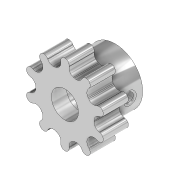
# Autodesk Inventor part: 4th Axis Main Drive Gear
Saved by Autodesk Inventor 2020 (Build 240168000, 168)
## iProperties
Created: 2021-06-28
Part Number: 4th Axis Main Drive Gear
Material: Generic
Document SubType Name: Modeling
Designer: Coy
Density: 1 g/cm^3
Appearance: Chrome - Polished
Author: Coy
Autodesk Inventor part; units mm, degrees
ref_plane "YZ Plane" through (0, 0, 0) normal (1, 0, 0) x (0, 1, 0)
ref_plane "XZ Plane" through (0, 0, 0) normal (0, 1, 0) x (-1, 0, 0)
ref_plane "XY Plane" through (0, 0, 0) normal (0, 0, 1) x (1, 0, 0)
sketch "Sketch4" plane through (0, 0, 0) normal (0, 0, 1) x (1, 0, 0)
  circle A0 centre (0, 0) radius 2.5
  circle A1 centre (0, 0) radius 8.2 construction
  arc A2 (1.0386, 6.9958) -> (-1.0386, 6.9958) centre (0, 7.15) ccw
  arc A3 (-1.7552, 5.7375) -> (-1.0238, 6.8958) centre (-2.0624, 6.7416) ccw
  arc A4 (1.0238, 6.8958) -> (1.7552, 5.7375) centre (2.0624, 6.7416) ccw
  line L0 (1.0238, 6.8958) -> (1.0386, 6.9958)
  line L1 (-1.0238, 6.8958) -> (-1.0386, 6.9958)
  line L2 (0, 0) -> (0, 6.1) construction
  line L3 (0, 8.2) -> (0, 9.5985) construction
  arc A5 (-3.2718, 6.2702) -> (-4.9523, 5.0492) centre (-4.2027, 5.7845) ccw
  line L4 (-4.8815, 4.9771) -> (-4.9523, 5.0492)
  arc A6 (-4.7924, 3.6101) -> (-4.8815, 4.9771) centre (-5.6311, 4.2418) ccw
  line L5 (-3.225, 6.1806) -> (-3.2718, 6.2702)
  arc A7 (-3.225, 6.1806) -> (-1.9524, 5.6734) centre (-2.2941, 6.6663) ccw
  arc A8 (-6.3325, 3.1496) -> (-6.9744, 1.174) centre (-6.8001, 2.2095) ccw
  line L6 (-6.8746, 1.1573) -> (-6.9744, 1.174)
  arc A9 (-5.9991, 0.1037) -> (-6.8746, 1.1573) centre (-7.0489, 0.1218) ccw
  line L7 (-6.2419, 3.1046) -> (-6.3325, 3.1496)
  arc A10 (-6.2419, 3.1046) -> (-4.9143, 3.4423) centre (-5.7743, 4.0447) ccw
  arc A11 (-6.9744, -1.174) -> (-6.3325, -3.1496) centre (-6.8001, -2.2095) ccw
  line L8 (-6.2419, -3.1046) -> (-6.3325, -3.1496)
  arc A12 (-4.9143, -3.4423) -> (-6.2419, -3.1046) centre (-5.7743, -4.0447) ccw
  line L9 (-6.8746, -1.1573) -> (-6.9744, -1.174)
  arc A13 (-6.8746, -1.1573) -> (-5.9991, -0.1037) centre (-7.0489, -0.1218) ccw
  arc A14 (-4.9523, -5.0492) -> (-3.2718, -6.2702) centre (-4.2027, -5.7845) ccw
  line L10 (-3.225, -6.1806) -> (-3.2718, -6.2702)
  arc A15 (-1.9524, -5.6734) -> (-3.225, -6.1806) centre (-2.2941, -6.6663) ccw
  line L11 (-4.8815, -4.9771) -> (-4.9523, -5.0492)
  arc A16 (-4.8815, -4.9771) -> (-4.7924, -3.6101) centre (-5.6311, -4.2418) ccw
  arc A17 (-1.0386, -6.9958) -> (1.0386, -6.9958) centre (0, -7.15) ccw
  line L12 (1.0238, -6.8958) -> (1.0386, -6.9958)
  arc A18 (1.7552, -5.7375) -> (1.0238, -6.8958) centre (2.0624, -6.7416) ccw
  line L13 (-1.0238, -6.8958) -> (-1.0386, -6.9958)
  arc A19 (-1.0238, -6.8958) -> (-1.7552, -5.7375) centre (-2.0624, -6.7416) ccw
  arc A20 (3.2718, -6.2702) -> (4.9523, -5.0492) centre (4.2027, -5.7845) ccw
  line L14 (4.8815, -4.9771) -> (4.9523, -5.0492)
  arc A21 (4.7924, -3.6101) -> (4.8815, -4.9771) centre (5.6311, -4.2418) ccw
  line L15 (3.225, -6.1806) -> (3.2718, -6.2702)
  arc A22 (3.225, -6.1806) -> (1.9524, -5.6734) centre (2.2941, -6.6663) ccw
  arc A23 (6.3325, -3.1496) -> (6.9744, -1.174) centre (6.8001, -2.2095) ccw
  line L16 (6.8746, -1.1573) -> (6.9744, -1.174)
  arc A24 (5.9991, -0.1037) -> (6.8746, -1.1573) centre (7.0489, -0.1218) ccw
  line L17 (6.2419, -3.1046) -> (6.3325, -3.1496)
  arc A25 (6.2419, -3.1046) -> (4.9143, -3.4423) centre (5.7743, -4.0447) ccw
  arc A26 (6.9744, 1.174) -> (6.3325, 3.1496) centre (6.8001, 2.2095) ccw
  line L18 (6.2419, 3.1046) -> (6.3325, 3.1496)
  arc A27 (4.9143, 3.4423) -> (6.2419, 3.1046) centre (5.7743, 4.0447) ccw
  line L19 (6.8746, 1.1573) -> (6.9744, 1.174)
  arc A28 (6.8746, 1.1573) -> (5.9991, 0.1037) centre (7.0489, 0.1218) ccw
  arc A29 (4.9523, 5.0492) -> (3.2718, 6.2702) centre (4.2027, 5.7845) ccw
  line L20 (3.225, 6.1806) -> (3.2718, 6.2702)
  arc A30 (1.9524, 5.6734) -> (3.225, 6.1806) centre (2.2941, 6.6663) ccw
  line L21 (4.8815, 4.9771) -> (4.9523, 5.0492)
  arc A31 (4.8815, 4.9771) -> (4.7924, 3.6101) centre (5.6311, 4.2418) ccw
  arc A32 (-1.7552, 5.7375) -> (-1.9524, 5.6734) centre (0, 0) ccw
  arc A33 (1.9524, 5.6734) -> (1.7552, 5.7375) centre (0, 0) ccw
  arc A34 (4.9143, 3.4423) -> (4.7924, 3.6101) centre (0, 0) ccw
  arc A35 (5.9991, -0.1037) -> (5.9991, 0.1037) centre (0, 0) ccw
  arc A36 (4.7924, -3.6101) -> (4.9143, -3.4423) centre (0, 0) ccw
  arc A37 (1.7552, -5.7375) -> (1.9524, -5.6734) centre (0, 0) ccw
  arc A38 (-1.9524, -5.6734) -> (-1.7552, -5.7375) centre (0, 0) ccw
  arc A39 (-4.9143, -3.4423) -> (-4.7924, -3.6101) centre (0, 0) ccw
  arc A40 (-4.7924, 3.6101) -> (-4.9143, 3.4423) centre (0, 0) ccw
  arc A41 (-5.9991, 0.1037) -> (-5.9991, -0.1037) centre (0, 0) ccw
  point P0 (-4.8198, 6.6339)
  point P1 (-7.7987, 2.5339)
  point P2 (-7.7987, -2.5339)
  point P3 (-4.8198, -6.6339)
  point P4 (0, -8.2)
  point P5 (4.8198, -6.6339)
  point P6 (7.7987, -2.5339)
  point P7 (7.7987, 2.5339)
  point P8 (4.8198, 6.6339)
  dimension "d19" = 5
  dimension "d20" = 16.4
  dimension "d22" = 2.1
  dimension "d23" = 2.1
  dimension "d24" = 2.1
  dimension "d27" = 360
  constraints: 90 point on circle, 44 end point, 42 centre point, 20 line through centre, 5 tangent, 2 coincident, 2 vertical, 151 other
  measures "d19" diameter of A0
  measures "d20" diameter of A1
  measures "d22" diameter of A2
  measures "d23" diameter of A4
  measures "d24" diameter of A3
extrude "Extrusion4" add sketch "Sketch4" along normal blind 5
sketch "Sketch5" plane through (0, 0, 0) normal (0, 0, -1) x (-1, 0, 0)
  circle A0 centre (0, 0) radius 2.5
  circle A1 centre (0, 0) radius 5.5
  dimension "d31" = 3
  constraints: 2 centre point, 1 coincident, 1 other
  measures "d31" radial gap between concentric circles of A0 A1
extrude "Extrusion5" add sketch "Sketch5" along normal blind 5
sketch "Sketch6" plane through (0, 0, 0) normal (1, 0, 0) x (0, 1, 0)
  line L0 (5.5, 0) -> (5.5, -5) projected
  line L1 (5.5, -2.5) -> (-5.5, -2.5) construction
  line L2 (-5.5, 0) -> (-5.5, -5) construction
  circle A0 centre (0, -2.5) radius 0.95
  point P0 (0, 0)
  dimension "d34" = 1.9
  constraints: 3 midpoint, 2 end point, 1 centre point
  measures "d34" diameter of A0
extrude "Extrusion6" cut sketch "Sketch6" against normal through all both and the other way through all
sketch "Sketch7" plane through (0, 0, 5) normal (0, 0, 1) x (1, 0, 0)
  arc A0 (-6.3325, 3.1496) -> (-6.9744, 1.174) centre (-6.8001, 2.2095) ccw projected
  line L0 (-6.9744, 1.174) -> (-6.8746, 1.1573) projected
  arc A1 (-5.9991, 0.1037) -> (-6.8746, 1.1573) centre (-7.0489, 0.1218) ccw projected
  arc A2 (-5.9991, 0.1037) -> (-5.9991, -0.1037) centre (0, 0) ccw projected
  arc A3 (-6.8746, -1.1573) -> (-5.9991, -0.1037) centre (-7.0489, -0.1218) ccw projected
  line L1 (-6.8746, -1.1573) -> (-6.9744, -1.174) projected
  arc A4 (-6.9744, -1.174) -> (-6.3325, -3.1496) centre (-6.8001, -2.2095) ccw projected
  line L2 (-6.3325, -3.1496) -> (-6.2419, -3.1046) projected
  arc A5 (-4.9143, -3.4423) -> (-6.2419, -3.1046) centre (-5.7743, -4.0447) ccw projected
  arc A6 (-4.9143, -3.4423) -> (-4.7924, -3.6101) centre (0, 0) ccw projected
  arc A7 (-4.8815, -4.9771) -> (-4.7924, -3.6101) centre (-5.6311, -4.2418) ccw projected
  line L3 (-4.8815, -4.9771) -> (-4.9523, -5.0492) projected
  arc A8 (-4.9523, -5.0492) -> (-3.2718, -6.2702) centre (-4.2027, -5.7845) ccw projected
  line L4 (-3.2718, -6.2702) -> (-3.225, -6.1806) projected
  arc A9 (-1.9524, -5.6734) -> (-3.225, -6.1806) centre (-2.2941, -6.6663) ccw projected
  arc A10 (-1.9524, -5.6734) -> (-1.7552, -5.7375) centre (0, 0) ccw projected
  arc A11 (-1.0238, -6.8958) -> (-1.7552, -5.7375) centre (-2.0624, -6.7416) ccw projected
  line L5 (-1.0238, -6.8958) -> (-1.0386, -6.9958) projected
  arc A12 (-1.0386, -6.9958) -> (1.0386, -6.9958) centre (0, -7.15) ccw projected
  line L6 (1.0386, -6.9958) -> (1.0238, -6.8958) projected
  arc A13 (1.7552, -5.7375) -> (1.0238, -6.8958) centre (2.0624, -6.7416) ccw projected
  arc A14 (1.7552, -5.7375) -> (1.9524, -5.6734) centre (0, 0) ccw projected
  arc A15 (3.225, -6.1806) -> (1.9524, -5.6734) centre (2.2941, -6.6663) ccw projected
  line L7 (3.225, -6.1806) -> (3.2718, -6.2702) projected
  arc A16 (3.2718, -6.2702) -> (4.9523, -5.0492) centre (4.2027, -5.7845) ccw projected
  line L8 (4.9523, -5.0492) -> (4.8815, -4.9771) projected
  arc A17 (4.7924, -3.6101) -> (4.8815, -4.9771) centre (5.6311, -4.2418) ccw projected
  arc A18 (4.7924, -3.6101) -> (4.9143, -3.4423) centre (0, 0) ccw projected
  arc A19 (6.2419, -3.1046) -> (4.9143, -3.4423) centre (5.7743, -4.0447) ccw projected
  line L9 (6.2419, -3.1046) -> (6.3325, -3.1496) projected
  arc A20 (6.3325, -3.1496) -> (6.9744, -1.174) centre (6.8001, -2.2095) ccw projected
  line L10 (6.9744, -1.174) -> (6.8746, -1.1573) projected
  arc A21 (5.9991, -0.1037) -> (6.8746, -1.1573) centre (7.0489, -0.1218) ccw projected
  arc A22 (5.9991, -0.1037) -> (5.9991, 0.1037) centre (0, 0) ccw projected
  arc A23 (6.8746, 1.1573) -> (5.9991, 0.1037) centre (7.0489, 0.1218) ccw projected
  line L11 (6.8746, 1.1573) -> (6.9744, 1.174) projected
  arc A24 (6.9744, 1.174) -> (6.3325, 3.1496) centre (6.8001, 2.2095) ccw projected
  line L12 (6.3325, 3.1496) -> (6.2419, 3.1046) projected
  arc A25 (4.9143, 3.4423) -> (6.2419, 3.1046) centre (5.7743, 4.0447) ccw projected
  arc A26 (4.9143, 3.4423) -> (4.7924, 3.6101) centre (0, 0) ccw projected
  arc A27 (4.8815, 4.9771) -> (4.7924, 3.6101) centre (5.6311, 4.2418) ccw projected
  line L13 (4.8815, 4.9771) -> (4.9523, 5.0492) projected
  arc A28 (4.9523, 5.0492) -> (3.2718, 6.2702) centre (4.2027, 5.7845) ccw projected
  line L14 (3.2718, 6.2702) -> (3.225, 6.1806) projected
  arc A29 (1.9524, 5.6734) -> (3.225, 6.1806) centre (2.2941, 6.6663) ccw projected
  arc A30 (1.9524, 5.6734) -> (1.7552, 5.7375) centre (0, 0) ccw projected
  arc A31 (1.0238, 6.8958) -> (1.7552, 5.7375) centre (2.0624, 6.7416) ccw projected
  line L15 (1.0238, 6.8958) -> (1.0386, 6.9958) projected
  arc A32 (1.0386, 6.9958) -> (-1.0386, 6.9958) centre (0, 7.15) ccw projected
  line L16 (-1.0386, 6.9958) -> (-1.0238, 6.8958) projected
  arc A33 (-1.7552, 5.7375) -> (-1.0238, 6.8958) centre (-2.0624, 6.7416) ccw projected
  arc A34 (-1.7552, 5.7375) -> (-1.9524, 5.6734) centre (0, 0) ccw projected
  arc A35 (-3.225, 6.1806) -> (-1.9524, 5.6734) centre (-2.2941, 6.6663) ccw projected
  line L17 (-3.225, 6.1806) -> (-3.2718, 6.2702) projected
  arc A36 (-3.2718, 6.2702) -> (-4.9523, 5.0492) centre (-4.2027, 5.7845) ccw projected
  line L18 (-4.9523, 5.0492) -> (-4.8815, 4.9771) projected
  arc A37 (-4.7924, 3.6101) -> (-4.8815, 4.9771) centre (-5.6311, 4.2418) ccw projected
  arc A38 (-4.7924, 3.6101) -> (-4.9143, 3.4423) centre (0, 0) ccw projected
  arc A39 (-6.2419, 3.1046) -> (-4.9143, 3.4423) centre (-5.7743, 4.0447) ccw projected
  line L19 (-6.2419, 3.1046) -> (-6.3325, 3.1496) projected
  circle A40 centre (0, 0) radius 2.5 projected
  arc A41 (-1.6967, 5.5463) -> (-1.8873, 5.4843) centre (0, 0) ccw
  arc A42 (-1.6967, 5.5463) -> (-0.8259, 6.9252) centre (-2.0624, 6.7416) ccw
  line L20 (-0.8259, 6.9252) -> (-0.8408, 7.0252)
  arc A43 (0.8408, 7.0252) -> (-0.8408, 7.0252) centre (0, 7.15) ccw
  line L21 (0.8408, 7.0252) -> (0.8259, 6.9252)
  arc A44 (0.8259, 6.9252) -> (1.6967, 5.5463) centre (2.0624, 6.7416) ccw
  arc A45 (1.8873, 5.4843) -> (1.6967, 5.5463) centre (0, 0) ccw
  arc A46 (1.8873, 5.4843) -> (3.4023, 6.088) centre (2.2941, 6.6663) ccw
  line L22 (3.4023, 6.088) -> (3.4491, 6.1777)
  arc A47 (4.8095, 5.1893) -> (3.4491, 6.1777) centre (4.2027, 5.7845) ccw
  line L23 (4.8095, 5.1893) -> (4.7387, 5.1171)
  arc A48 (4.7387, 5.1171) -> (4.6327, 3.4897) centre (5.6311, 4.2418) ccw
  arc A49 (4.7505, 3.3276) -> (4.6327, 3.4897) centre (0, 0) ccw
  arc A50 (4.7505, 3.3276) -> (6.331, 2.9255) centre (5.7743, 4.0447) ccw
  line L24 (6.331, 2.9255) -> (6.4215, 2.9705)
  arc A51 (6.9412, 1.3713) -> (6.4215, 2.9705) centre (6.8001, 2.2095) ccw
  line L25 (6.9412, 1.3713) -> (6.8414, 1.3545)
  arc A52 (6.8414, 1.3545) -> (5.7991, 0.1002) centre (7.0489, 0.1218) ccw
  arc A53 (5.7991, -0.1002) -> (5.7991, 0.1002) centre (0, 0) ccw
  arc A54 (5.7991, -0.1002) -> (6.8414, -1.3545) centre (7.0489, -0.1218) ccw
  line L26 (6.8414, -1.3545) -> (6.9412, -1.3713)
  arc A55 (6.4215, -2.9705) -> (6.9412, -1.3713) centre (6.8001, -2.2095) ccw
  line L27 (6.4215, -2.9705) -> (6.331, -2.9255)
  arc A56 (6.331, -2.9255) -> (4.7505, -3.3276) centre (5.7743, -4.0447) ccw
  arc A57 (4.6327, -3.4897) -> (4.7505, -3.3276) centre (0, 0) ccw
  arc A58 (4.6327, -3.4897) -> (4.7387, -5.1171) centre (5.6311, -4.2418) ccw
  line L28 (4.7387, -5.1171) -> (4.8095, -5.1893)
  arc A59 (3.4491, -6.1777) -> (4.8095, -5.1893) centre (4.2027, -5.7845) ccw
  line L29 (3.4491, -6.1777) -> (3.4023, -6.088)
  arc A60 (3.4023, -6.088) -> (1.8873, -5.4843) centre (2.2941, -6.6663) ccw
  arc A61 (1.6967, -5.5463) -> (1.8873, -5.4843) centre (0, 0) ccw
  arc A62 (1.6967, -5.5463) -> (0.8259, -6.9252) centre (2.0624, -6.7416) ccw
  line L30 (0.8259, -6.9252) -> (0.8408, -7.0252)
  arc A63 (-0.8408, -7.0252) -> (0.8408, -7.0252) centre (0, -7.15) ccw
  line L31 (-0.8408, -7.0252) -> (-0.8259, -6.9252)
  arc A64 (-0.8259, -6.9252) -> (-1.6967, -5.5463) centre (-2.0624, -6.7416) ccw
  arc A65 (-1.8873, -5.4843) -> (-1.6967, -5.5463) centre (0, 0) ccw
  arc A66 (-1.8873, -5.4843) -> (-3.4023, -6.088) centre (-2.2941, -6.6663) ccw
  line L32 (-3.4023, -6.088) -> (-3.4491, -6.1777)
  arc A67 (-4.8095, -5.1893) -> (-3.4491, -6.1777) centre (-4.2027, -5.7845) ccw
  line L33 (-4.8095, -5.1893) -> (-4.7387, -5.1171)
  arc A68 (-4.7387, -5.1171) -> (-4.6327, -3.4897) centre (-5.6311, -4.2418) ccw
  arc A69 (-4.7505, -3.3276) -> (-4.6327, -3.4897) centre (0, 0) ccw
  arc A70 (-4.7505, -3.3276) -> (-6.331, -2.9255) centre (-5.7743, -4.0447) ccw
  line L34 (-6.331, -2.9255) -> (-6.4215, -2.9705)
  arc A71 (-6.9412, -1.3713) -> (-6.4215, -2.9705) centre (-6.8001, -2.2095) ccw
  line L35 (-6.9412, -1.3713) -> (-6.8414, -1.3545)
  arc A72 (-6.8414, -1.3545) -> (-5.7991, -0.1002) centre (-7.0489, -0.1218) ccw
  arc A73 (-5.7991, 0.1002) -> (-5.7991, -0.1002) centre (0, 0) ccw
  arc A74 (-5.7991, 0.1002) -> (-6.8414, 1.3545) centre (-7.0489, 0.1218) ccw
  line L36 (-6.8414, 1.3545) -> (-6.9412, 1.3713)
  arc A75 (-6.4215, 2.9705) -> (-6.9412, 1.3713) centre (-6.8001, 2.2095) ccw
  line L37 (-6.4215, 2.9705) -> (-6.331, 2.9255)
  arc A76 (-6.331, 2.9255) -> (-4.7505, 3.3276) centre (-5.7743, 4.0447) ccw
  arc A77 (-4.6327, 3.4897) -> (-4.7505, 3.3276) centre (0, 0) ccw
  arc A78 (-4.6327, 3.4897) -> (-4.7387, 5.1171) centre (-5.6311, 4.2418) ccw
  line L38 (-4.7387, 5.1171) -> (-4.8095, 5.1893)
  arc A79 (-3.4491, 6.1777) -> (-4.8095, 5.1893) centre (-4.2027, 5.7845) ccw
  line L39 (-3.4491, 6.1777) -> (-3.4023, 6.088)
  arc A80 (-3.4023, 6.088) -> (-1.8873, 5.4843) centre (-2.2941, 6.6663) ccw
  circle A81 centre (0, 0) radius 2.7
  dimension "d24" = 2.1
  dimension "d27" = 360
  dimension "d42" = 0.2
  dimension "d43" = 0.2
  constraints: 80 point on circle, 41 centre point, 40 end point, 59 other
  measures "d42" radial gap between concentric circles of A35 A80
  measures "d43" radial gap between concentric circles of A40 A81
extrude "Extrusion7" cut sketch "Sketch7" against normal blind 25.4
chamfer "Chamfer2" distance 7 angle 2 1 edges at (-2.7, 0, -5) measured on face at (-2.7, 0, -4.5)
fillet "Fillet3" radius 0.3 5 edges at (-2.9444, 0, -5) (5.4173, -0.95, -2.5001) (-5.4173, -0.95, -2.4999) (-5.4549, 0.703, -3.139) (-5.4549, 0.703, -1.861)
equation "\"d23\" = d22"
equation "\"d24\" = d22"
body "Solid2"
